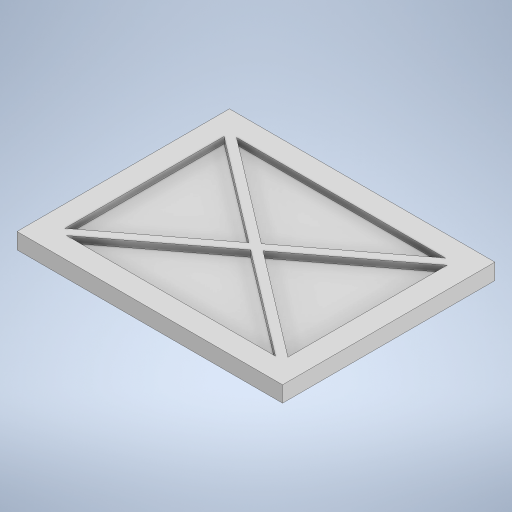
# Autodesk Inventor part: planeDerzavki
Saved by Autodesk Inventor 2024 (Build 280153000, 153)
## iProperties
Created: 2023-09-10
Part Number: planeDerzavki
Material: Generic
Document SubType Name: Modeling
Designer: KirikDK
Density: 1 g/cm^3
Appearance: Default
Author: KirikDK
Autodesk Inventor part; units mm, degrees
ref_plane "YZ Plane" through (0, 0, 0) normal (1, 0, 0) x (0, 1, 0)
ref_plane "XZ Plane" through (0, 0, 0) normal (0, 1, 0) x (-1, 0, 0)
ref_plane "XY Plane" through (0, 0, 0) normal (0, 0, 1) x (1, 0, 0)
sketch "Sketch1" plane through (0, 0, 0) normal (0, 1, 0) x (-1, 0, 0)
  line L0 (66.6667, 111.1111) -> (-183.3333, 111.1111)
  line L1 (-183.3333, 111.1111) -> (-183.3333, -88.8889)
  line L2 (-183.3333, -88.8889) -> (66.6667, -88.8889)
  line L3 (66.6667, -88.8889) -> (66.6667, 111.1111)
  point P0 (0, 0)
  dimension "d0" = 200
  dimension "d1" = 250
  constraints: 8 end point, 2 parallel, 1 horizontal, 1 perpendicular
  measures "d0" distance of L2.end L0.start
  measures "d1" distance of L0.start L0.end
extrude "Extrusion1" add sketch "Sketch1" along normal blind 15
sketch "Sketch2" plane through (0, 15, 0) normal (0, 1, 0) x (1, 0, 0)
  line L0 (183.3333, -111.1111) -> (183.3333, 88.8889) projected
  line L1 (183.3333, 88.8889) -> (-66.6667, 88.8889) projected
  line L2 (-66.6667, 88.8889) -> (-66.6667, -111.1111) projected
  line L3 (-66.6667, -111.1111) -> (183.3333, -111.1111) projected
  line L4 (-46.6667, -91.1111) -> (-46.6667, 68.8889)
  line L5 (-46.6667, 68.8889) -> (163.3333, 68.8889)
  line L6 (163.3333, 68.8889) -> (163.3333, -91.1111)
  line L7 (163.3333, -91.1111) -> (-46.6667, -91.1111)
  line L8 (-46.6667, -91.1111) -> (163.3333, 68.8889)
  line L9 (163.3333, -91.1111) -> (-46.6667, 68.8889)
  line L10 (160.9092, -94.2928) -> (-49.0908, 65.7072)
  line L11 (165.7575, -87.9294) -> (-44.2425, 72.0706)
  line L12 (-49.0908, -87.9294) -> (160.9092, 72.0706)
  line L13 (-44.2425, -94.2928) -> (165.7575, 65.7072)
  point P0 (0, 0)
  point P1 (58.3333, -16.1398)
  point P2 (-40.0665, -91.1111)
  point P3 (156.7331, -91.1111)
  point P4 (163.3333, 63.8602)
  point P5 (64.9335, -11.1111)
  point P6 (163.3333, -86.0824)
  point P7 (58.3333, -6.0824)
  point P8 (156.7331, 68.8889)
  point P9 (-40.0665, 68.8889)
  point P10 (-46.6667, -86.0824)
  point P11 (51.7331, -11.1111)
  point P12 (-46.6667, 63.8602)
  dimension "d4" = 20
  dimension "d5" = 4
  dimension "d6" = 4
  dimension "d7" = 4
  dimension "d8" = 4
  constraints: 20 end point, 4 parallel, 3 other
  measures "d4" distance between parallel lines of L2 L4
  measures "d5" distance between parallel lines of L12 L8
  measures "d6" distance between parallel lines of L13 L8
  measures "d7" distance between parallel lines of L11 L9
  measures "d8" distance between parallel lines of L10 L9
extrude "Extrusion2" cut sketch "Sketch2" against normal blind 6 contours L4 L10 L12 | L13 L10 L7 | L5 L12 L11 | L11 L13 L6
body "Solid1"
